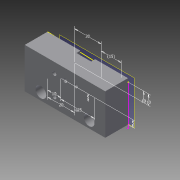
# Autodesk Inventor part: detalKKoretke
Saved by Autodesk Inventor 2015 (Build 190159000, 159)
## iProperties
Created: 2016-04-08
Part Number: detalKKoretke
Material: Generic
Document SubType Name: Modeling
Designer: Andreas
Density: 1 g/cm^3
Appearance: Default
Author: Andreas
Autodesk Inventor part; units mm, degrees
ref_plane "YZ Plane" through (0, 0, 0) normal (1, 0, 0) x (0, 1, 0)
ref_plane "XZ Plane" through (0, 0, 0) normal (0, 1, 0) x (-1, 0, 0)
ref_plane "XY Plane" through (0, 0, 0) normal (0, 0, 1) x (1, 0, 0)
sketch "Sketch1" plane through (0, 0, 0) normal (0, 1, 0) x (-1, 0, 0)
  line L0 (0, 2.5) -> (60, 2.5)
  line L1 (60, 2.5) -> (60, -27.5)
  line L2 (60, -27.5) -> (0, -27.5)
  line L3 (0, -27.5) -> (0, 2.5)
  dimension "d0" = 60
  dimension "d1" = 30
  dimension "d2" = 60
  dimension "d164" = 90
  dimension "d165" = 90
  constraints: 8 end point, 1 coincident
  measures "d0" distance of L0.start L0.end
  measures "d1" distance of L0.end L1.end
  measures "d2" distance of L1.end L2.end
  measures "d164" angle of L0 L3
  measures "d165" angle of L3 L2
extrude "Extrusion1" add sketch "Sketch1" against normal blind 5 and the other way blind 12
sketch "Sketch2" plane through (0, 12, 0) normal (0, 1, 0) x (1, 0, 0)
  line L0 (-60, 27.5) -> (-60, -2.5) projected
  line L1 (0, 0) -> (0, 30) projected
  line L2 (0, 27.5) -> (-60, 27.5) projected
  line L3 (-60, -2.5) -> (0, -2.5) projected
  line L4 (-5, 0) -> (-5, 30) projected
  point P0 (-40, 7.5)
  point P1 (-20, 7.5)
  dimension "d44" = 10
  dimension "d45" = 20
  dimension "d46" = 20
  dimension "d47" = 10
  dimension "d67" = 15
  constraints: 2 other
  measures "d45" distance from line of L0 point (-40, 7.5)
  measures "d46" distance of point (-40, 7.5) point (-20, 7.5)
  measures "d67" distance from line of L4 point (-20, 7.5)
sketch "Sketch3" plane through (0, 12, 0) normal (0, 1, 0) x (1, 0, 0)
  line L0 (0, 27.5) -> (-60, 27.5) projected
  line L1 (-60, -2.5) -> (-60, 27.5) projected
  point P0 (0, 0)
  point P1 (-50, 22.5)
  point P2 (-5, 30)
  point P3 (-25, 22.5)
  dimension "d56" = 5
  dimension "d57" = 10
  dimension "d58" = 25
  dimension "d59" = 5
  constraints: 1 other
  measures "d57" distance from line of L1 point (-50, 22.5)
  measures "d58" distance of point (-50, 22.5) point (-25, 22.5)
sketch "Sketch16" plane through (-60, -5, 2.5) normal (0, 0, 1) x (1, 0, 0)
  line L0 (60, 17) -> (0, 17) projected
  line L1 (24.5, 16.25) -> (24.5, 14)
  line L2 (24.5, 14) -> (35.5, 14)
  line L3 (35.5, 14) -> (35.5, 16.25)
  line L4 (35.5, 17) -> (24.5, 17)
  line L5 (60, 0) -> (0, 0) projected
  line L6 (0, 17) -> (60, 17) projected
  line L7 (24.5, 16.25) -> (24.5, 17)
  line L8 (35.5, 17) -> (35.5, 16.25)
  point P0 (60, 5)
  point P1 (25.5, 17)
  point P2 (30, 17)
  point P3 (30, 0)
  point P4 (30, 17)
  point P5 (30, 0)
  point P6 (30, 17)
  point P7 (30, 0)
  dimension "d90" = 1
  dimension "d92" = 2.25
  dimension "d93" = 11
  constraints: 12 end point, 6 midpoint, 4 point on line, 3 perpendicular, 3 vertical alignment, 1 parallel
  measures "d90" distance of L4.end point (25.5, 17)
  measures "d92" distance of L1.start L1.end
  measures "d93" distance of L1.end L2.end
extrude "Extrusion6" cut sketch "Sketch16" against normal up to next
sketch "Sketch17" plane through (-35.5, 9, 2.5) normal (0, 1, 0) x (1, 0, 0)
  circle A0 centre (5.5, 8) radius 1.5
  line L0 (0, 30) -> (11, 30) projected
  line L1 (11, 0) -> (0, 0) projected
  point P0 (35.5, 2.5)
  point P1 (5.5, 30)
  dimension "d97" = 3
  dimension "d155" = 8
  constraints: 1 centre point, 1 midpoint, 1 vertical alignment
  measures "d97" diameter of A0
  measures "d155" distance from line of L1 A0.centre
extrude "Extrusion7" cut sketch "Sketch17" against normal up to next
ref_plane "Work Plane2" through (0, 15.5, 0) normal (0, 1, 0) x (1, 0, 0)
sketch "Sketch21" plane through (0, -5, 0) normal (0, -1, 0) x (1, 0, 0)
  circle A0 centre (-12, -22) radius 4
  circle A1 centre (-48, -22) radius 4
  point P0 (0, 0)
  dimension "d125" = 8
  dimension "d131" = 8
  constraints: 2 centre point
  measures "d125" diameter of A0
  measures "d131" diameter of A1
extrude "Extrusion13" cut sketch "Sketch21" against normal blind 12
sketch "Sketch23" plane through (-12, 7, -22) normal (0, -1, 0) x (1, 0, 0)
  circle A0 centre (0, 0) radius 1.5
  circle A1 centre (-36, 0) radius 1.5
  point P0 (12, 22)
  dimension "d134" = 3
  dimension "d135" = 3
  constraints: 2 centre point
  measures "d134" diameter of A0
  measures "d135" diameter of A1
extrude "Extrusion14" cut sketch "Sketch23" against normal up to next
sketch "Sketch25" plane through (0, 12, 0) normal (0, 1, 0) x (1, 0, 0)
  circle A0 centre (-22, 5) radius 1.5
  circle A1 centre (-22, 20) radius 1.5
  circle A2 centre (-38, 20) radius 1.5
  circle A3 centre (-38, 5) radius 1.5
  line L0 (-60, -2.5) -> (0, -2.5) projected
  line L1 (-60, 27.5) -> (-60, -2.5) projected
  point P0 (0, 0)
  point P1 (-34.5, 0)
  dimension "d145" = 3
  dimension "d146" = 3
  dimension "d147" = 3
  dimension "d148" = 3
  dimension "d149" = 16
  dimension "d150" = 15
  dimension "d151" = 7.5
  dimension "d152" = 22
  constraints: 4 centre point, 2 horizontal alignment, 2 vertical alignment, 1 other
  measures "d145" diameter of A0
  measures "d146" diameter of A1
  measures "d147" diameter of A2
  measures "d148" diameter of A3
  measures "d149" distance of A3.centre A0.centre
  measures "d150" distance of A1.centre A0.centre
  measures "d152" distance from line of L1 A3.centre
extrude "Extrusion16" cut sketch "Sketch25" against normal up to next
sketch "Sketch26" plane through (0, 12, 0) normal (0, 1, 0) x (1, 0, 0)
  circle A0 centre (-38, 20) radius 3
  circle A1 centre (-22, 20) radius 3
  circle A2 centre (-38, 5) radius 3
  circle A3 centre (-22, 5) radius 3
  line L0 (-60, -2.5) -> (-35.5, -2.5) projected
  point P0 (0, 0)
  dimension "d156" = 6
  dimension "d157" = 6
  dimension "d160" = 6
  dimension "d161" = 6
  dimension "d166" = 15
  dimension "d167" = 16
  dimension "d168" = 7.5
  constraints: 4 centre point, 2 horizontal alignment, 2 vertical alignment
  measures "d156" diameter of A0
  measures "d157" diameter of A1
  measures "d160" diameter of A2
  measures "d161" diameter of A3
  measures "d166" distance of A2.centre A0.centre
  measures "d167" distance of A1.centre A0.centre
  measures "d168" distance from line of L0 A2.centre
extrude "Extrusion18" cut sketch "Sketch26" against normal blind 8
sketch "Sketch11" plane through (0, 12, 0) normal (0, 1, 0) x (1, 0, 0)
  point P0 (-20, 10)
  point P1 (-40, 10)
body "Solid1"
